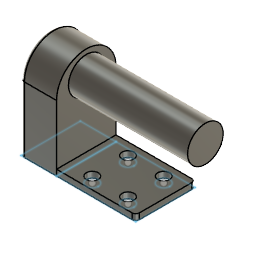
2nd (Autodesk Fusion 360 design; units mm, degrees)
part number: 2026-07-24-20-53-34-395
Autodesk Fusion 360 part; units mm, degrees
sketch "Sketch3" plane through (0, 0, 0) normal (0, 0, 1) x (1, 0, 0)
  circle A0 centre (-250, 150) radius 5
  circle A1 centre (-220, 150) radius 5
  circle A2 centre (-250, 120) radius 5
  circle A3 centre (-220, 120) radius 5
  line L0 (-270, 160) -> (-203.4896, 160)
  line L1 (-203.4896, 160) -> (-203.4896, 110)
  line L2 (-203.4896, 110) -> (-270, 110)
  line L3 (-270, 110) -> (-270, 160)
  line L4 (-270, 160) -> (-300, 160)
  line L5 (-300, 160) -> (-300, 110)
  line L6 (-300, 110) -> (-270, 110)
  line L7 (-270, 110) -> (-270, 160)
  dimension "d13" = 10
  dimension "d14" = 10
  dimension "d15" = 10
  dimension "d16" = 10
  constraint horizontal L0
  constraint vertical L1
  constraint horizontal L2
  constraint vertical L3
  constraint horizontal L4
  constraint vertical L5
  constraint horizontal L6
  constraint vertical L7
  constraint coincident L3 L0.start
  measures "d13" diameter of A3
  measures "d14" diameter of A2
  measures "d15" diameter of A0
  measures "d16" diameter of A1
extrude "Extrude1" add sketch "Sketch3" along normal blind 5 contours L0 L1 L2 L3 L7
extrude "Extrude2" add sketch "Sketch3" along normal blind 80 contours L3 L4 L5 L6 L7
sketch "Sketch6" plane through (-270, 0, 0) normal (1, 0, 0) x (0, 1, 0)
  line L0 (110, 5) -> (160, 5)
  line L1 (160, 5) -> (160, 80)
  line L2 (160, 80) -> (110, 80)
  line L3 (110, 80) -> (110, 0)
  circle A0 centre (135, 61) radius 15
  line L4 (110, 0) -> (110, 0)
  line L5 (110, 0) -> (110, 5)
  dimension "d6" = 30
  measures "d6" diameter of A0
extrude "Extrude3" add sketch "Sketch6" along normal blind 100 contours A0
fillet "Fillet1" radius 25 2 edges at (-285, 160, 80) (-285, 110, 80)
fillet "Fillet3" radius 3 5 edges at (-203.4896, 160, 2.5) (-203.4896, 110, 2.5) (-300, 110, 27.5) (-300, 135, 80) (-300, 160, 27.5)
